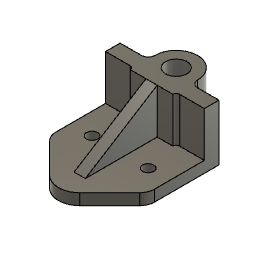
A3 v3 (Autodesk Fusion 360 design; units mm, degrees)
Autodesk Fusion 360 part; units mm, degrees
sketch "Base" plane through (0, 0, 0) normal (0, 1, 0) x (1, 0, 0)
  line L0 (44, 33.5) -> (-44, 33.5)
  line L1 (44, -10.9853) -> (44, 33.5)
  line L2 (44, 33.5) -> (-44, -33.5) construction
  line L3 (-44, 33.5) -> (44, -33.5) construction
  line L4 (-44, 33.5) -> (44, 33.5)
  line L5 (44, 33.5) -> (44, 30.5)
  line L6 (-44, 30.5) -> (-44, 33.5)
  line L7 (-44, 30.5) -> (-40.0597, 30.5)
  line L8 (-44, -10.9853) -> (-44, 30.5)
  line L9 (44, -10.9853) -> (44, 30.5)
  arc A0 (-13.435, -46.935) -> (13.435, -46.935) centre (0, -33.5) ccw
  line L10 (0, -33.5) -> (-13.435, -46.935) construction
  line L11 (0, -33.5) -> (13.435, -46.935) construction
  line L12 (-13.435, -46.935) -> (-40.1924, -20.1777)
  line L13 (13.435, -46.935) -> (40.1924, -20.1777)
  line L14 (-44, 33.5) -> (-44, -10.9853)
  arc A1 (40.1924, -20.1777) -> (44, -10.9853) centre (31, -10.9853) ccw
  arc A2 (-44, -10.9853) -> (-40.1924, -20.1777) centre (-31, -10.9853) ccw
  line L15 (-44, 33.5) -> (44, 33.5)
  line L16 (44, 33.5) -> (44, 2.5)
  line L17 (-44, 2.5) -> (-44, 33.5)
  line L18 (0, 33.5) -> (-25, 33.5)
  line L19 (-25, -33.5) -> (0, -33.5) construction
  line L20 (0, -33.5) -> (25, -33.5) construction
  line L21 (25, 33.5) -> (0, 33.5)
  circle A3 centre (-25, 2.5) radius 5
  circle A4 centre (25, 2.5) radius 5
  line L22 (-44, 33.5) -> (44, 33.5)
  line L23 (44, 33.5) -> (44, 46.5)
  line L24 (-44, 46.5) -> (-44, 33.5)
  line L25 (-44, 46.5) -> (-25, 46.5)
  line L26 (-19, 33.5) -> (-44, 33.5)
  line L27 (-44, 33.5) -> (-44, 46.5)
  line L28 (44, 46.5) -> (25, 46.5)
  line L29 (19, 33.5) -> (44, 33.5)
  line L30 (44, 33.5) -> (44, 46.5)
  line L31 (44, 46.5) -> (44, 52.5) construction
  line L32 (44, 52.5) -> (-44, 52.5) construction
  line L33 (-44, 52.5) -> (-44, 46.5) construction
  circle A5 centre (0, 52.5) radius 9.5
  arc A6 (-25, 46.5) -> (-19, 52.5) centre (-25, 52.5) ccw
  arc A7 (19, 52.5) -> (25, 46.5) centre (25, 52.5) ccw
  arc A8 (19, 52.5) -> (-19, 52.5) centre (0, 52.5) ccw
  line L34 (-44, 46.5) -> (-25, 46.5)
  line L35 (25, 46.5) -> (44, 46.5)
  line L36 (44, 46.5) -> (25, 46.5)
  line L37 (-25, 46.5) -> (-44, 46.5)
  dimension "d1" = 88
  dimension "d2" = 67
  dimension "d3" = 3
  dimension "d6" = 38
  dimension "d10" = 13
  dimension "d11" = 31
  dimension "d12" = 25
  dimension "d13" = 25
  dimension "d14" = 10
  dimension "d15" = 10
  dimension "d38" = 13
  dimension "d43" = 6
  dimension "d44" = 19
  dimension "d45" = 38
  dimension "d46" = 6
  dimension "d47" = 6
  constraint horizontal L0
  constraint perpendicular L0 L14
  constraint parallel L1 L14
  constraint coincident L2 origin
  constraint coincident L3 origin
  constraint horizontal L4
  constraint vertical L5
  constraint vertical L6
  constraint horizontal L7
  constraint vertical L8
  constraint vertical L9
  constraint coincident A0.centre L10.start
  constraint perpendicular L10 L11
  constraint tangent A0 L12
  constraint tangent L8 A2
  constraint tangent L12 A2
  constraint horizontal L15
  constraint vertical L16
  constraint vertical L17
  constraint horizontal L18
  constraint horizontal L19
  constraint midpoint L4 L18.start
  constraint horizontal L20
  constraint horizontal L21
  constraint coincident L3 L7.end
  constraint horizontal L22
  constraint vertical L23
  constraint horizontal L36
  constraint vertical L24
  constraint horizontal L25
  constraint horizontal L26
  constraint vertical L27
  constraint horizontal L28
  constraint horizontal L29
  constraint vertical L30
  constraint horizontal L34
  constraint vertical L31
  constraint horizontal L32
  constraint vertical L33
  constraint midpoint L32 A5.centre
  constraint concentric A5 A8
  constraint tangent A6 L34
  constraint tangent A7 L34
  constraint coincident L32 A6.end
  constraint coincident L25.end L36
  constraint coincident L32 A7.start
  constraint collinear L34 L35
  constraint collinear L36 L37
  measures "d1" distance of L2.end L3.end
  measures "d2" distance of L0.end L2.end
  measures "d3" distance of L0.end L6.start
  measures "d6" diameter of A0
  measures "d10" radius of A2
  measures "d11" distance of L0.end L17.start
  measures "d12" distance of L18.start L18.end
  measures "d13" distance of A0.centre L20.end
  measures "d14" diameter of A3
  measures "d15" diameter of A4
  measures "d38" distance of L0.end L24.start
  measures "d43" distance of L24.start L32.end
  measures "d44" diameter of A5
  measures "d45" diameter of A8
  measures "d46" radius of A6
  measures "d47" radius of A7
extrude "Extrude1" add sketch "Base" along normal blind 10 contours L0 L1 L4 L5 L6 L8 L9 A0 L12 L13 L14 A1 A2 L15 L16 L17 L18 L21 L22 L26 L29
sketch "Base decorations" plane through (0, 10, 0) normal (0, 1, 0) x (-1, 0, 0)
  circle A0 centre (-25, -2.5) radius 5
  circle A1 centre (25, -2.5) radius 5
  line L0 (-44, -33.5) -> (44, -33.5)
  line L1 (44, -33.5) -> (44, 10.9853)
  arc A2 (44, 10.9853) -> (40.1924, 20.1777) centre (31, 10.9853) ccw
  line L2 (40.1924, 20.1777) -> (13.435, 46.935)
  arc A3 (13.435, 46.935) -> (-13.435, 46.935) centre (0, 33.5) ccw
  line L3 (-13.435, 46.935) -> (-40.1924, 20.1777)
  arc A4 (-40.1924, 20.1777) -> (-44, 10.9853) centre (-31, 10.9853) ccw
  line L4 (-44, 10.9853) -> (-44, -33.5)
  line L5 (44, -33.5) -> (-44, -33.5)
  line L6 (-44, -33.5) -> (-44, -30.5)
  line L7 (44, -30.5) -> (44, -33.5)
  line L8 (44, -30.5) -> (19, -30.5)
  line L9 (44, 10.5) -> (44, -30.5)
  line L10 (-44, -30.5) -> (-19, -30.5)
  line L11 (-44, 10.5) -> (-44, -30.5)
  line L12 (19, -30.5) -> (5, -30.5)
  line L13 (5, -30.5) -> (5, 10.5)
  line L14 (-19, -30.5) -> (-5, -30.5)
  line L15 (-5, -30.5) -> (-5, 10.5)
  line L16 (-5, -30.5) -> (-5, -26.5)
  line L17 (-5, -26.5) -> (5, -26.5)
  line L18 (5, -26.5) -> (5, -30.5)
  line L19 (5, -33.5) -> (-5, -33.5)
  line L20 (-5, -30.5) -> (-5, 33.5)
  line L21 (-5, 33.5) -> (5, 33.5)
  line L22 (5, 33.5) -> (5, -30.5)
  line L23 (-44, -30.5) -> (-5, -30.5)
  line L24 (5, -30.5) -> (44, -30.5)
  line L25 (19, -30.5) -> (5, -30.5)
  line L26 (-5, -30.5) -> (-19, -30.5)
  line L27 (44, -33.5) -> (19, -33.5)
  line L28 (19, -30.5) -> (44, -30.5)
  line L29 (44, -30.5) -> (44, -33.5)
  line L30 (-44, -33.5) -> (-19, -33.5)
  line L31 (-19, -30.5) -> (-44, -30.5)
  line L32 (-44, -30.5) -> (-44, -33.5)
  arc A5 (-22, -33.5) -> (-19, -30.5) centre (-22, -30.5) ccw
  arc A6 (19, -30.5) -> (22, -33.5) centre (22, -30.5) ccw
  dimension "d18" = 3
  dimension "d19" = 25
  dimension "d20" = 41
  dimension "d21" = 25
  dimension "d22" = 41
  dimension "d23" = 14
  dimension "d24" = 14
  dimension "d26" = 4
  dimension "d27" = 67
  dimension "d28" = 25
  dimension "d29" = 25
  dimension "d30" = 3
  dimension "d31" = 3
  constraint horizontal L5
  constraint vertical L6
  constraint horizontal L23
  constraint vertical L7
  constraint coincident L0.end L1.start
  constraint horizontal L8
  constraint vertical L9
  constraint horizontal L10
  constraint vertical L11
  constraint horizontal L25
  constraint horizontal L12
  constraint vertical L13
  constraint horizontal L14
  constraint vertical L15
  constraint vertical L16
  constraint horizontal L17
  constraint vertical L18
  constraint horizontal L19
  constraint vertical L20
  constraint horizontal L21
  constraint vertical L22
  constraint coincident L5 L19.start
  constraint collinear L23 L24
  constraint collinear L25 L26
  constraint horizontal L27
  constraint horizontal L28
  constraint vertical L29
  constraint horizontal L30
  constraint horizontal L31
  constraint vertical L32
  constraint tangent L27 A6
  constraint tangent L5 A5
  constraint coincident L0 A5.start
  constraint coincident L0 A6.end
  measures "d18" distance of L0.end L7.start
  measures "d19" distance of L7.start L8.end
  measures "d20" distance of L7.start L9.start
  measures "d21" distance of L6.end L10.end
  measures "d22" distance of L6.end L11.start
  measures "d23" distance of L8.end L12.end
  measures "d24" distance of L10.end L14.end
  measures "d26" distance of L12.end L17.end
  measures "d27" distance of L19.start L21.end
  measures "d28" distance of L0.end L27.end
  measures "d29" distance of L0.start L30.end
  measures "d30" radius of A6
  measures "d31" radius of A5
extrude "Extrude4" add sketch "Base decorations" along normal blind 40 contours L0 L5 L12 L13 L14 L15 L16 L17 L18 L19 L20 L22 L23 L24 L25 L26 L27 L30 A5 A6
extrude "Extrude2" add sketch "Base decorations" along normal blind 40 contours L13 L15 L17 L20 L21 L22
sketch "Triangle cut" plane through (5, 0, 0) normal (1, 0, 0) x (0, 0, -1)
  line L0 (-33.5, 10) -> (30.5, 10)
  line L1 (30.5, 50) -> (-33.5, 50)
  line L2 (-33.5, 50) -> (-33.5, 10)
  line L3 (30.5, 50) -> (-33.5, 10)
  line L4 (30.5, 10) -> (30.5, 50)
  constraint coincident L1.start L3.start
  constraint coincident L0.start L2.end
extrude "Extrude3" cut sketch "Triangle cut" against normal blind 10 contours L1 L2 L3
extrude "Extrude5" add sketch "Base" along normal blind 50 contours L0 L4 L15 L18 L21 L22 L23 L24 L25 L26 L27 L28 L29 L30 A6 A7 A8 L34 L35 L36 L37
